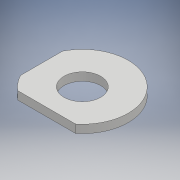
# Autodesk Inventor part: shayba
Saved by Autodesk Inventor 2018.2 (Build 222227000, 227)
## iProperties
Created: 2026-01-20
Part Number: shayba
Material: Типовые
Document SubType Name: Modeling
Designer: Denis
Density: 1 g/cm^3
Appearance: По умолчанию
Author: Denis
## iProperties of the stored document shayba_3DПЕЧАТЬ.ipt
Created: 2026-01-20
Part Number: shayba_3DПЕЧАТЬ
Material: Типовые
Document SubType Name: Modeling
Designer: Denis
Density: 1 g/cm^3
Appearance: По умолчанию
Author: Denis
Autodesk Inventor part; units mm, degrees
ref_plane "YZ Plane" through (0, 0, 0) normal (1, 0, 0) x (0, 1, 0)
ref_plane "XZ Plane" through (0, 0, 0) normal (0, 1, 0) x (-1, 0, 0)
ref_plane "XY Plane" through (0, 0, 0) normal (0, 0, 1) x (1, 0, 0)
sketch "Эскиз1" plane through (0, 0, 0) normal (0, 0, 1) x (1, 0, 0)
  circle A0 centre (0, 0) radius 4.5
  dimension "d0" = 9
  constraints: 1 centre point, 1 coincident
  measures "d0" diameter of A0
extrude "Выдавливание1" add sketch "Эскиз1" along normal blind 0.8
sketch "Эскиз2" plane through (0, 0, 0.8) normal (0, 0, 1) x (1, 0, 0)
  circle A0 centre (0, 0) radius 1.8
  dimension "d3" = 3.6
  constraints: 1 centre point, 1 coincident
  measures "d3" diameter of A0
extrude "Выдавливание2" cut sketch "Эскиз2" against normal blind 0.8
sketch "Эскиз3" plane through (0, 0, 0.8) normal (0, 0, 1) x (1, 0, 0)
  line L0 (0, 0) -> (0, -3.5)
  line L1 (0, 0) -> (-4, 0)
  circle A0 centre (0, 0) radius 4.5 projected
  line L2 (-4, -2.0616) -> (-5.2131, -2.0616)
  line L3 (-5.2131, -2.0616) -> (-5.2131, 3.1786)
  line L4 (-5.2131, 3.1786) -> (-4, 3.1786)
  line L5 (-4, 3.1786) -> (-4, -2.0616)
  line L6 (-2.8284, -3.5) -> (4.77, -3.5)
  line L7 (4.77, -3.5) -> (4.77, -5.6057)
  line L8 (4.77, -5.6057) -> (-2.8284, -5.6057)
  line L9 (-2.8284, -5.6057) -> (-2.8284, -3.5)
  dimension "d6" = 3.5
  dimension "d7" = 4
  constraints: 20 end point, 4 parallel, 3 horizontal, 2 perpendicular, 2 point on circle, 1 vertical
  measures "d6" distance of L0.start L0.end
  measures "d7" distance of L0.start L1.end
extrude "Выдавливание3" cut sketch "Эскиз3" against normal blind 10 contours L6 A0 | L5 A0 | A0 L6 L7 L8 L9 | L2 L3 L4 L5 A0
